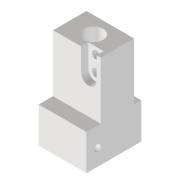
# Autodesk Inventor part: 40_XYZstage_micrometer_motorized_nema8_nanotec_adapter_z
Saved by Autodesk Inventor 2022 (Build 260153000, 153)
## iProperties
Created: 2023-04-17
Part Number: 40_XYZstage_micrometer_motorized_nema8_nanotec_adapter_z
Material: Generisch
Document SubType Name: Modeling
Designer: diederichbenedict
Density: 1 g/cm^3
Appearance: Vorgabe
Author: diederichbenedict
Autodesk Inventor part; units mm, degrees
ref_plane "YZ Plane" through (0, 0, 0) normal (1, 0, 0) x (0, 1, 0)
ref_plane "XZ Plane" through (0, 0, 0) normal (0, 1, 0) x (-1, 0, 0)
ref_plane "XY Plane" through (0, 0, 0) normal (0, 0, 1) x (1, 0, 0)
sketch "Skizze6" plane through (0, 0, 0) normal (0, 0, 1) x (1, 0, 0)
  line L0 (0, 0) -> (-20, 0)
  line L1 (-20, 0) -> (-20, 24)
  line L2 (-20, 24) -> (0, 24)
  line L3 (0, 24) -> (0, 0)
  circle A0 centre (-5, 21) radius 1.65
  circle A1 centre (-5, 14.5) radius 1.65
  dimension "d29" = 20
  dimension "d30" = 24
  dimension "d31" = 3.3
  dimension "d32" = 3.3
  dimension "d33" = 3
  dimension "d34" = 6.5
  dimension "d35" = 5
  constraints: 8 end point, 2 centre point, 2 parallel, 1 horizontal, 1 perpendicular
  measures "d29" distance of L1.end L2.end
  measures "d30" distance of L0.end L1.end
  measures "d31" diameter of A0
  measures "d32" diameter of A1
  measures "d33" vertical distance of A0.centre L2.end
  measures "d34" distance of A1.centre A0.centre
  measures "d35" distance from line of A0.centre L3
extrude "Extrusion5" add sketch "Skizze6" along normal blind 14
sketch "Skizze7" plane through (-20, 0, 0) normal (0, -1, 0) x (1, 0, 0)
  line L0 (0, 0) -> (20, 0) projected
  line L1 (20, 0) -> (20, 14) projected
  line L2 (0, 14) -> (20, 14) projected
  line L3 (0, 0) -> (0, 14) projected
  circle A0 centre (10, 7) radius 4
  dimension "d38" = 8
  dimension "d39" = 10
  constraints: 1 centre point
  measures "d38" diameter of A0
  measures "d39" distance from line of A0.centre L3
extrude "Extrusion6" cut sketch "Skizze7" against normal through all contours A0
sketch "Skizze8" plane through (0, 0, 14) normal (0, 0, 1) x (1, 0, 0)
  line L0 (0, 24) -> (-20, 24) projected
  line L1 (-20, 24) -> (-20, 0) projected
  line L2 (-20, 0) -> (0, 0) projected
  line L3 (0, 0) -> (0, 24) projected
  circle A0 centre (-5, 14.5) radius 1.65 projected
  circle A1 centre (-5, 21) radius 1.65 projected
  line L4 (-5, 14.5) -> (-5, 31.6413) construction
  line L5 (-1.75, 14.5) -> (-1.75, 31.6413)
  line L6 (-8.25, 31.6413) -> (-8.25, 14.5)
  arc A2 (-8.25, 14.5) -> (-1.75, 14.5) centre (-5, 14.5) ccw
  arc A3 (-1.75, 31.6413) -> (-8.25, 31.6413) centre (-5, 31.6413) ccw
  point P0 (-5, 23.0707)
  dimension "d42" = 6.5
  constraints: 8 end point, 4 point on circle, 4 tangent, 2 centre point, 1 midpoint, 1 parallel, 1 vertical
  measures "d42" diameter of A3
extrude "Extrusion7" cut sketch "Skizze8" against normal blind 3 contours L5 A2 L6 L0 | L0 L6 A3 L5 | A0 | A1
sketch "Skizze9" plane through (-20, 0, 0) normal (0, -1, 0) x (1, 0, 0)
  circle A0 centre (10, 7) radius 4 projected
  line L0 (0, 0) -> (20, 0) projected
  line L1 (20, 0) -> (20, 14) projected
  line L2 (0, 14) -> (20, 14) projected
  line L3 (0, 0) -> (0, 14) projected
  circle A1 centre (10, 7) radius 7.25
  line L4 (20, 17) -> (0, 17)
  line L5 (0, 17) -> (0, -3)
  line L6 (0, -3) -> (20, -3)
  line L7 (20, -3) -> (20, 17)
  line L8 (20, 17) -> (0, -3) construction
  line L9 (0, 17) -> (20, -3) construction
  line L10 (0, 17) -> (20, 17)
  line L11 (20, 17) -> (20, 20)
  line L12 (20, 20) -> (0, 20)
  line L13 (0, 20) -> (0, 17)
  dimension "d45" = 14.5
  dimension "d46" = 20
  dimension "d47" = 20
  dimension "d50" = 3
  constraints: 20 end point, 4 parallel, 2 horizontal, 2 midpoint, 2 perpendicular, 1 centre point, 1 coincident
  measures "d45" diameter of A1
  measures "d46" distance of L6.end L5.end
  measures "d47" distance of L5.end L4.end
  measures "d50" distance of L11.end L10.end
extrude "Extrusion8" add sketch "Skizze9" along normal blind 15 contours L3 L2 A1 L0 | L0 A1 L7 L6 L5 | L5 L4 L7 L2 A1 | A1 L2 L1 L0 | L13 L12 L11 L4
sketch "Skizze10" plane through (-20, 24, 0) normal (-1, 0, 0) x (0, 0, 1)
  line L0 (14.25, -39) -> (14.25, -24) projected
  circle A0 centre (15.3846, -32.1377) radius 1.4
  point P0 (0, -24)
  dimension "d51" = 2.8
  constraints: 1 centre point
  measures "d51" diameter of A0
hole "Bohrung2" at (-20, -8.1377, 15.3846) direction (1, 0, 0) diameter 2.8 end through all counterbore diameter 6.5 counterbore depth 4
